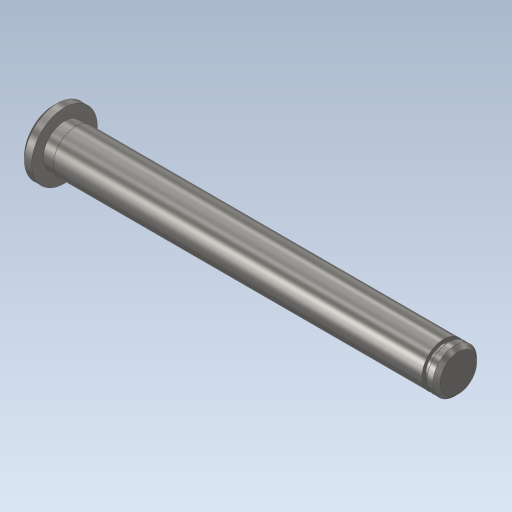
# Autodesk Inventor part: GSHCCGH6-52.0_D
Saved by Autodesk Inventor 2024 (Build 280153000, 153)
## iProperties
Category: PARTsolutions
Company: MISUMI
Created: 2023-10-14
Part Number: GSHCCGH6-52.0_D
Material: ステンレス鋼
Catalog Web Link: www.cadenas.de
Description: HCCG, HCCGH, PHCCG, PHCCGH, GHCCH, SHCCG, SHCCGH, GSHCCGH_D-Hinge Pins - Retaining Ring Type with Shoulder - L Dimension Specified Type (0.1mm Increment)
Vendor: MISUMI
Document SubType Name: Modeling
Designer: psAdmin
Manufacturer: MISUMI
Mass: 7.86478 g
Surface Area: 9.56692 cm^2
Volume: 0.983097 cm^3
Density: 8 g/cm^3
Appearance: 半つや出し
PSOL_IDENT_0: {$CADENAS_DATA/23d-libs/misumi/metric/13_cantilever_shafts/hccg_d.prj},275 {VTYP=3D},{NB=GSHCCGH6-52
PSOL_IDENT_1: .0_D},{LINA=GSHCCGH6-52.0},{NN=HCCG, HCCGH, PHCCG, PHCCGH, GHCCH, SHCCG, SHCCGH, GSHCCGH_D},{DATE=21
PSOL_IDENT_2: .04.2022 08:37:14},{GEOMDATE=16.06.2021 01:26:14},{VERSION=},{LINEID=40},{WBVAR=MAT,HARD,ST,L,ALT1,N
PSOL_IDENT_3: C,ALT2,TC,ALT3,ALT4,TBH},{WBNUMERIC=L,NC,TC,TBH}  {NB=GSHCCGH6-52.0_D},{LINA=GSHCCGH6-52.0},{KT=DUMM
PSOL_IDENT_4: Y},{PN=GSHCCGH6-52.0},{TYPE=GSHCCGH},{MAT=3},{HARD=5},{HARD1= '4','45~50HRC','5','45~50HRC Plating H
PSOL_IDENT_5: ardness 750HV~' },{ST=4},{ST1='4','Hard Chrome Plating'},{AC=Retaining Ring 1 pc.},{MATAC=SUS304},{D=
PSOL_IDENT_6: 6},{DTOL=-0.004/-0.012},{L=52.0},{LS1=[5.0-120.0/0.1]},{L2=52},{L3=0},{LPN=52.0},{M=0.70},{MTOL=+0.1
PSOL_IDENT_7: /0},{ALT1=},{NC=0.0},{N=2},{N1=2},{NC1=[1.9-4.0/0.1]},{NC2=0},{NC3=0},{NC4=0},{NCPN=0.0},{ALT1PN=},{
PSOL_IDENT_8: UU=5.8},{NN=1.5},{DD=5.0},{DDTOL=+0.075/0},{ALT2=},{TC=0.0},{T=1.5},{TT1=1.5},{TC1=0},{TC2=0},{TC3=0
PSOL_IDENT_9: },{TCPN=0.0},{ALT2PN=},{H=9.0},{RRS=E Type},{RRN=5},{RRNC=0.000},{ALT3=},{HC=3.50},{RMAT=-S},{RMATC=
PSOL_IDENT_10: -S},{ALT4=},{ALT4ALG= '', 'w/o TBH (Shoulder Diameter)', '-TBH', 'with TBH (Shoulder Diameter)' },{T
PSOL_IDENT_11: BH=0},{TBHALG=0},{TBHMIN=7.0},{TBHMAX=8.5},{H3D=9.0},{ALT4PN=}
NB: GSHCCGH6-52.0_D
NN: 1.5
NT: Hinge Pins - Retaining Ring Type with Shoulder - L Dimension Specified Type (0.1mm Increment)
NBSYN: $PN._D
LINA: GSHCCGH6-52.0
CATALOG: Misumi
PN: GSHCCGH6-52.0
MAT: SUS440C or 13Cr Stainless Steel
HARD: 45~50HRC Plating Hardness 750HV~
ST: Hard Chrome Plating
MATAC: SUS304
D: 6
L: 52
M: 0.7
MTOL: +0.1/0
ALT1: w/o NC (Retaining Ring Groove Position)
NC: 0
N: 2
UU: 5.8
DD: 5
DDTOL: +0.075/0
ALT2: w/o TC (Shoulder Thickness)
TC: 0
T: 1.5
H: 9
RRS: E Type
RRN: 5
RRNC: 0
ALT3: w/o HC (Shoulder Diameter Cut)
ALT4: w/o TBH (Shoulder Diameter)
TBH: 0
SUPPLIER: MISUMI
ARTICLENO: GSHCCGH6-52.0_D
BOMINFO: GSHCCGH6-52.0
CREATOR: CADENAS GmbH
Title: GSHCCGH6-52.0
Author: Cadenas PARTsolutions
Comments: Hinge Pins - Retaining Ring Type with Shoulder - L Dimension Specified Type (0.1mm Increment)
Autodesk Inventor part; units mm, degrees
sketch "Sketch_1" plane through (0, 0, 0) normal (0, 0, 1) x (1, 0, 0)
  line L0 (55.5, 0) -> (0, 0)
  line L1 (0, 0) -> (0, 4)
  line L2 (0, 4) -> (0.5, 4.5)
  line L3 (0.5, 4.5) -> (1.5, 4.5)
  line L4 (1.5, 4.5) -> (1.5, 2.9)
  line L5 (1.5, 2.9) -> (3, 2.9)
  line L6 (3, 2.9) -> (3, 3)
  line L7 (3, 3) -> (53.5, 3)
  line L8 (53.5, 3) -> (53.5, 2.5)
  line L9 (53.5, 2.5) -> (54.2, 2.5)
  line L10 (54.2, 2.5) -> (54.2, 3)
  line L11 (54.2, 3) -> (55, 3)
  line L12 (55, 3) -> (55.5, 2.5)
  line L13 (55.5, 2.5) -> (55.5, 0)
  line L14 (55.5, 0) -> (0, 0)
  constraints: 30 end point
revolve "Revolution1" add sketch "Sketch_1" angle 360 about axis through (55.5, 0, 0) along (1, 0, 0)
ref_plane "pin_to_body_XY" through (1.5, 0, 0) normal (1, 0, 0) x (0, 0, -1)
ref_plane "pin_to_body_YZ" through (1.5, 0, 0) normal (0, 0, -1) x (0, 1, 0)
ref_plane "pin_to_body_ZX" through (1.5, 0, 0) normal (0, 1, 0) x (1, 0, 0)
ref_plane "pin_to_knuckle_XY" through (27.5, 0, 0) normal (-1, 0, 0) x (0, 0, -1)
ref_plane "pin_to_knuckle_YZ" through (27.5, 0, 0) normal (0, 0, -1) x (0, -1, 0)
ref_plane "pin_to_knuckle_ZX" through (27.5, 0, 0) normal (0, -1, 0) x (-1, 0, 0)
ref_plane "pin_to_rring_XY" through (53.85, 0, 0) normal (-1, 0, 0) x (0, 0, -1)
ref_plane "pin_to_rring_YZ" through (53.85, 0, 0) normal (0, 0, -1) x (0, -1, 0)
ref_plane "pin_to_rring_ZX" through (53.85, 0, 0) normal (0, -1, 0) x (-1, 0, 0)
body "Solid1"
